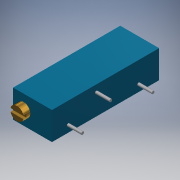
# Autodesk Inventor part: RES-PRESET-3006P
Saved by Autodesk Inventor 2018.3 (Build 223284000, 284)
## iProperties
Created: 2021-03-26
Part Number: RES-PRESET-3006P
Material: Genérico
Document SubType Name: Modeling
Designer: laguerre
Density: 8.47 g/cm^3
Appearance: Valor por defecto
Author: laguerre
Autodesk Inventor part; units mm, degrees
ref_plane "YZ Plane" through (0, 0, 0) normal (1, 0, 0) x (0, 1, 0)
ref_plane "XZ Plane" through (0, 0, 0) normal (0, 1, 0) x (-1, 0, 0)
ref_plane "XY Plane" through (0, 0, 0) normal (0, 0, 1) x (1, 0, 0)
sketch "Boceto39" plane through (0, 0, 0) normal (0, 0, 1) x (1, 0, 0)
  circle A0 centre (0, 1.27) radius 0.25
  circle A1 centre (5.08, -1.27) radius 0.25
  circle A2 centre (-7.62, -1.27) radius 0.25
  point P0 (0, 0)
  dimension "d373" = 0.5
  dimension "d374" = 1.27
  dimension "d375" = 2.54
  dimension "d376" = 12.7
  dimension "d377" = 5.08
  constraints: 3 centre point, 2 equal radius, 1 horizontal alignment, 1 vertical alignment
  measures "d373" diameter of A2
  measures "d374" distance of A0.centre point (0, 0)
  measures "d375" vertical distance of A0.centre A1.centre
  measures "d376" distance of A1.centre A2.centre
  measures "d377" horizontal distance of A1.centre A0.centre
extrude "Extrusión13" add sketch "Boceto39" against normal blind 2.6
sketch "Boceto40" plane through (0, 0, 0) normal (0, 0, 1) x (1, 0, 0)
  line L0 (-11.3, 2.5) -> (8, 2.5)
  line L1 (8, 2.5) -> (8, -2.5)
  line L2 (8, -2.5) -> (-11.3, -2.5)
  line L3 (-11.3, -2.5) -> (-11.3, 2.5)
  point P0 (0, 0)
  point P1 (8, 0)
  dimension "d380" = 5
  dimension "d381" = 19.3
  dimension "d382" = 8
  constraints: 8 end point, 2 parallel, 1 horizontal, 1 horizontal alignment, 1 midpoint, 1 perpendicular
  measures "d380" distance of L0.end L1.end
  measures "d381" distance of L0.start L0.end
  measures "d382" distance from line of point (0, 0) L1
extrude "Extrusión14" add sketch "Boceto40" along normal blind 7
sketch "Boceto41" plane through (8, -2.5, 0) normal (1, 0, 0) x (0, 0, -1)
  circle A0 centre (-5.1, 2.5) radius 1.2
  line L0 (-7, 0) -> (-7, 5) projected
  line L1 (0, 5) -> (0, 0) projected
  point P0 (0, 2.5)
  point P1 (0, 2.5)
  dimension "d385" = 2.4
  dimension "d386" = 1.9
  constraints: 1 centre point, 1 horizontal alignment, 1 midpoint
  measures "d385" diameter of A0
  measures "d386" distance from line of A0.centre L0
extrude "Extrusión15" add sketch "Boceto41" along normal blind 1.2
sketch "Boceto42" plane through (9.2, 0, 5.1) normal (1, 0, 0) x (0, 0, -1)
  line L0 (-1.4485, 0.3) -> (1.5656, 0.3)
  line L1 (1.5656, 0.3) -> (1.5656, -0.3)
  line L2 (1.5656, -0.3) -> (-1.4485, -0.3)
  line L3 (-1.4485, -0.3) -> (-1.4485, 0.3)
  point P0 (5.1, 0)
  point P1 (1.5656, 0)
  dimension "d389" = 0.6
  constraints: 8 end point, 2 parallel, 1 horizontal, 1 horizontal alignment, 1 midpoint, 1 perpendicular
  measures "d389" distance between parallel lines of L2 L0
extrude "Extrusión16" cut sketch "Boceto42" against normal blind 0.5
